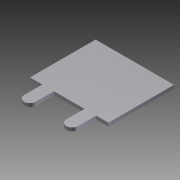
# Autodesk Inventor part: M201230TX-switch
Saved by Autodesk Inventor 2011 SP1 (Build 150282100, 282)
## iProperties
Created: 2013-12-24
Part Number: M201230TX-switch
Catalog Web Link: www.cadenas.de
Description: Angle Mount Miniature Rockers - Shroud Terminals-Series M - Miniature Rockers
Vendor: NKKSWITCHES
Document SubType Name: Modeling
Designer: PARTuser1
Manufacturer: NKKSWITCHES
Density: 1 g/cm^3
Category: PARTsolutions
Company: NKKSWITCHES
Title: M201230TX-switch
Author: Cadenas PARTsolutions
Comments: Series M - Miniature Rockers
PSOL_IDENT_0: {$CADENAS_DATA\23d-libs\nkkswitches\toggle\m\parts\m_ang_t_shroudterm.prj},236 {VTYP=3D},{NB=M201230
PSOL_IDENT_1: TX-switch},{LINA=M201230TX-switch},{NN=Angle Mount Miniature Rockers - Shroud Terminals},{DATE=28.05
PSOL_IDENT_2: .2007 07:27:48},{GEOMDATE=28.05.2007 00:00:00},{VERSION=},{LINEID=10},{LINESUBID=-1},{WBVAR=PLS,CRCT
PSOL_IDENT_3: S,FRM,TRMNLS}  {NB=M201230TX-switch},{LINA=M201230TX-switch},{KT=DUMMY},{PN=M201230TX},{SRS=M20},{PL
PSOL_IDENT_4: S=1},{CRCTSALG='2','2 - ON/NONE/ON','3','3 - ON/OFF/ON','5','5 - ON/NONE/(ON)','8','8 - (ON)/OFF/(ON
PSOL_IDENT_5: )','9','9 - ON/OFF/(ON)','4', '4 - ON/ON/ON','6','6 - (ON)/ON/(ON)','7','7 - ON/ON/(ON)'},{CRCTS=2},
PSOL_IDENT_6: {FRMALG='TX', 'TX - Narrow Frame for Small Actuator', 'TZ'  , 'TZ - Wide Frame for Large Actuator'},
PSOL_IDENT_7: {FRM=TX},{TRMNLSALG='30', '30 - .150\" (3.81mm) Right Angle PC (1-3 Pole)', '32'  , '32 -  Right Ang
PSOL_IDENT_8: le PCB (1 Pole & 0.4VA Rating Only', '40'  , '40 - .150\" (3.81mm) Vertical PC (1-4 Pole)', '45'  ,
PSOL_IDENT_9: '45 - .100\" (2.54mm) Vertical PC (1-4 Pole)'},{TRMNLS=30},{WIDTH=0.512},{HEIGHT=0.3877},{LENGTH=0.3
PSOL_IDENT_10: 11},{A=0.15},{TRMNLNOH=1},{TRMNLOV=3},{LTRMNL=0.031},{POS=0},{POS2=0.185},{POS3=0},{D=0},{HOLES=0.18
PSOL_IDENT_11: 5},{WH=0.00000},{D1=0.00000},{D2=0.00000}
CNS_NN: Angle Mount Miniature Rockers - Shroud Terminals
CNS_NT: Series M - Miniature Rockers
CNS_NB: M201230TX-switch
CNS_NBSYN: $PN.-switch
CNS_LINA: M201230TX-switch
CNS_PN: M201230TX
CNS_SRS: M20
CNS_PLS: 1 - SPST/SPDT
CNS_CRCTSALG: '2','2 - ON/NONE/ON','3','3 - ON/OFF/ON','5','5 - ON/NONE/(ON)','8','8 - (ON)/OFF/(ON)','9','9 - ON/OFF/(ON)','4', '4 - ON/ON/ON','6','6 - (ON)/ON/(ON)','7','7 - ON/ON/(ON)'
CNS_CRCTS: 2 - ON/NONE/ON
CNS_FRMALG: 'TX', 'TX - Narrow Frame for Small Actuator', 'TZ'  , 'TZ - Wide Frame for Large Actuator'
CNS_FRM: TX - Narrow Frame for Small Actuator
CNS_TRMNLSALG: '30', '30 - .150" (3.81mm) Right Angle PC (1-3 Pole)', '32'  , '32 -  Right Angle PCB (1 Pole & 0.4VA Rating Only', '40'  , '40 - .150" (3.81mm) Vertical PC (1-4 Pole)', '45'  , '45 - .100" (2.54mm) Vertical PC (1-4 Pole)'
CNS_TRMNLS: 30 - .150" (3.81mm) Right Angle PC (1-3 Pole)
CNS_WIDTH: 0.512
CNS_HEIGHT: 0.388
CNS_LENGTH: 0.311
CNS_A: 0.150
CNS_TRMNLNOH: 1.000
CNS_TRMNLOV: 3.000
CNS_LTRMNL: 0.031
CNS_POS: 0.000
CNS_POS2: 0.185
CNS_POS3: 0.000
CNS_D: 0.000
CNS_HOLES: 0.185
CNS_WH: 0.00000
CNS_D1: 0.00000
CNS_D2: 0.00000
SUPPLIER: NKKSWITCHES
ARTICLENO: M201230TX-switch
BOMINFO: M201230TX-switch
CREATOR: CADENAS GmbH
Autodesk Inventor part; units mm, degrees
sketch "Sketch_1" plane through (0, 0, 0) normal (0, 1, 0) x (-1, 0, 0)
  line L0 (4.7244, 3.9497) -> (3.2385, 3.9497)
  line L1 (3.2385, 3.9497) -> (3.2385, 6.1468)
  arc A0 (3.2385, 6.1468) -> (1.8415, 6.1468) centre (2.54, 6.1468) ccw
  line L2 (1.8415, 6.1468) -> (1.8415, 3.9497)
  line L3 (1.8415, 3.9497) -> (-1.8415, 3.9497)
  line L4 (-1.8415, 3.9497) -> (-1.8415, 6.1468)
  arc A1 (-1.8415, 6.1468) -> (-3.2385, 6.1468) centre (-2.54, 6.1468) ccw
  line L5 (-3.2385, 6.1468) -> (-3.2385, 3.9497)
  line L6 (-3.2385, 3.9497) -> (-4.7244, 3.9497)
  line L7 (-4.7244, 3.9497) -> (-4.7244, -3.9497)
  line L8 (-4.7244, -3.9497) -> (4.7244, -3.9497)
  line L9 (4.7244, -3.9497) -> (4.7244, 3.9497)
  constraints: 20 end point, 4 point on circle, 2 centre point
extrude "Extrusion1" add sketch "Sketch_1" along normal blind 0.4064
ref_plane "shtrmnl_XY" through (0, 0, 0) normal (0, 1, 0) x (1, 0, 0)
ref_plane "shtrmnl_YZ" through (0, 0, 0) normal (1, 0, 0) x (0, 0, -1)
ref_plane "shtrmnl_ZX" through (0, 0, 0) normal (0, 0, -1) x (0, 1, 0)
body "Solid1"
